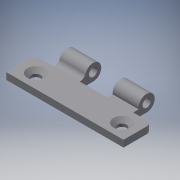
# Autodesk Inventor part: hinge_v1
Saved by Autodesk Inventor 2019 (Build 230136000, 136)
## iProperties
Created: 2020-12-01
Part Number: hinge_v1
Material: Generic
Document SubType Name: Modeling
Designer: close
Density: 1 g/cm^3
Appearance: Default
Author: close
Autodesk Inventor part; units mm, degrees
ref_plane "YZ Plane" through (0, 0, 0) normal (1, 0, 0) x (0, 1, 0)
ref_plane "XZ Plane" through (0, 0, 0) normal (0, 1, 0) x (-1, 0, 0)
ref_plane "XY Plane" through (0, 0, 0) normal (0, 0, 1) x (1, 0, 0)
sketch "Sketch1" plane through (0, 0, 0) normal (1, 0, 0) x (0, 1, 0)
  line L0 (0, 0) -> (2.5, 0)
  line L1 (2.5, 0) -> (2.5, -12.642)
  line L2 (0, -15.6) -> (0, 0)
  arc A0 (0, -15.6) -> (2.5, -12.642) centre (3, -15.6) ccw
  circle A1 centre (3, -15.6) radius 1.55
  point P0 (2.5, -5.2)
  dimension "d0" = 3
  dimension "d1" = 3.1
  dimension "d2" = 2.5
  dimension "d3" = 5.2
  dimension "d4" = 10.4
  dimension "d5" = 3
  constraints: 6 end point, 2 centre point, 2 point on circle, 1 coincident, 1 horizontal, 1 parallel, 1 perpendicular, 1 point on line
  measures "d0" radius of A0
  measures "d1" diameter of A1
  measures "d2" distance between parallel lines of L2 L1
  measures "d3" distance from line of L0 point (2.5, -5.2)
  measures "d4" vertical distance of A0.centre point (2.5, -5.2)
  measures "d5" distance from line of L2 A0.centre
extrude "Extrusion1" add sketch "Sketch1" along normal blind 43.5
sketch "Sketch2" plane through (0, 0, -15.6) normal (0, -1, 0) x (1, 0, 0)
  line L0 (0, -3) -> (43.5, -3) projected
  line L1 (26.875, -3) -> (16.625, -3)
  line L2 (16.625, -3) -> (16.625, 5)
  line L3 (16.625, 5) -> (26.875, 5)
  line L4 (26.875, 5) -> (26.875, -3)
  line L5 (43.5, -3) -> (43.5, 3) projected
  line L6 (43.5, -3) -> (36.5, -3)
  line L7 (36.5, -3) -> (36.5, 5)
  line L8 (36.5, 5) -> (43.5, 5)
  line L9 (43.5, 5) -> (43.5, -3)
  line L10 (0, -3) -> (7, -3)
  line L11 (7, -3) -> (7, 5)
  line L12 (7, 5) -> (0, 5)
  line L13 (0, 5) -> (0, -3)
  line L14 (43.5, 15.6) -> (43.5, 0) projected
  point P0 (0, 15.6)
  point P1 (43.5, 2.958)
  dimension "d8" = 10.25
  dimension "d9" = 43.5
  dimension "d10" = 16.625
  dimension "d11" = 8
  dimension "d12" = 7
  dimension "d13" = 7
  constraints: 24 end point, 6 parallel, 3 horizontal, 3 perpendicular, 2 point on line, 1 collinear
  measures "d8" distance between parallel lines of L2 L4
  measures "d9" distance between parallel lines of L13 L14
  measures "d10" distance between parallel lines of L4 L5
  measures "d11" distance between parallel lines of L0 L3
  measures "d12" distance between parallel lines of L14 L7
  measures "d13" distance between parallel lines of L13 L11
extrude "Extrusion2" cut sketch "Sketch2" against normal through all
sketch "Sketch3" plane through (0, 2.5, 0) normal (0, 1, 0) x (1, 0, 0)
  line L0 (0, 5.2) -> (43.5, 5.2) construction
  line L1 (43.5, 10.6) -> (43.5, 0) construction
  point P0 (0, 0)
  point P1 (5.75, 5.2)
  point P2 (37.75, 5.2)
  dimension "d16" = 32
  dimension "d17" = 43.5
  dimension "d18" = 5.75
  constraints: 3 point on line, 2 end point, 1 horizontal
  measures "d16" distance of point (37.75, 5.2) point (5.75, 5.2)
  measures "d17" distance from line of point (0, 0) L1
  measures "d18" horizontal distance of point (5.75, 5.2) point (0, 0)
hole "Hole1" at (5.75, 2.5, -5.2) at (37.75, 2.5, -5.2) direction (0, -1, 0) diameter 3.4 depth 2.5 countersink diameter 6.3 countersink angle 90 clearance for "Flat Head Machine Screw" size "M3" standard "Ansi Metric M Profile"
fillet "Fillet1" radius 2 3 edges at (0, 1.25, -10.6) (43.5, 1.25, -10.6) (11.8125, 2.5, -12.642)
equation "\"d5\" = d0"
equation "\"d10\" = -0.5 * d8 + 0.5 * d9"
equation "\"d13\" = d12"
equation "\"d18\" = -0.5 * d16 + 0.5 * d17"
body "Solid1"
